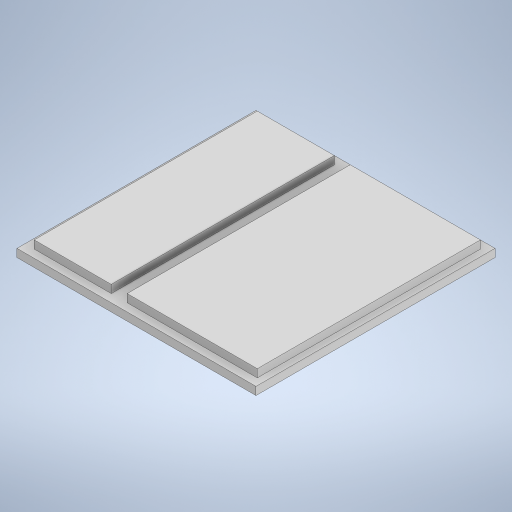
# Autodesk Inventor part: víčko
Saved by Autodesk Inventor 2024 (Build 280153000, 153)
## iProperties
Created: 2025-04-21
Part Number: víčko
Material: Všeobecné
Document SubType Name: Modeling
Designer: annav
Density: 1 g/cm^3
Appearance: Výchozí
Author: ANNA VÁVROVÁ
Autodesk Inventor part; units mm, degrees
ref_plane "YZ Plane" through (0, 0, 0) normal (1, 0, 0) x (0, 1, 0)
ref_plane "XZ Plane" through (0, 0, 0) normal (0, 1, 0) x (-1, 0, 0)
ref_plane "XY Plane" through (0, 0, 0) normal (0, 0, 1) x (1, 0, 0)
sketch "Náčrt1" plane through (0, 0, 0) normal (0, 1, 0) x (-1, 0, 0)
  line L0 (0, -63) -> (0, 63) projected
  line L1 (-63, 0) -> (63, 0) projected
  line L2 (45, 45) -> (-45, 45)
  line L3 (-45, 45) -> (-45, -45)
  line L4 (-45, -45) -> (45, -45)
  line L5 (45, -45) -> (45, 45)
  point P0 (0, 0)
  dimension "d0" = 90
  dimension "d1" = 90
  constraints: 8 end point, 2 parallel, 1 horizontal, 1 perpendicular, 2 other
  measures "d0" distance of L2.end L3.end
  measures "d1" distance between parallel lines of L3 L5
extrude "Vysunutí1" add sketch "Náčrt1" along normal blind 3
sketch "Náčrt2" plane through (0, 3, 0) normal (0, 1, 0) x (1, 0, 0)
  line L0 (0, 63) -> (0, -63) projected
  line L1 (63, 0) -> (-63, 0) projected
  line L2 (-41.5, -42) -> (-12.5, -42)
  line L3 (-12.5, -42) -> (-12.5, 42)
  line L4 (-12.5, 42) -> (-41.5, 42)
  line L5 (-41.5, 42) -> (-41.5, -42)
  line L6 (-45, 45) -> (-45, -45) projected
  point P0 (0, 0)
  dimension "d4" = 3.5
  dimension "d5" = 29
  dimension "d6" = 84
  constraints: 8 end point, 2 parallel, 1 horizontal, 1 perpendicular, 1 other
  measures "d4" distance between parallel lines of L5 L6
  measures "d5" distance between parallel lines of L3 L5
  measures "d6" distance between parallel lines of L4 L2
extrude "Vysunutí2" add sketch "Náčrt2" along normal blind 3
sketch "Náčrt3" plane through (0, 3, 0) normal (0, 1, 0) x (1, 0, 0)
  line L0 (-12.5, -42) -> (-12.5, 42) projected
  line L1 (0, 63) -> (0, -63) projected
  line L2 (63, 0) -> (-63, 0) projected
  line L3 (-6.5, -42) -> (42.5, -42)
  line L4 (42.5, -42) -> (42.5, 42)
  line L5 (42.5, 42) -> (-6.5, 42)
  line L6 (-6.5, 42) -> (-6.5, -42)
  point P0 (0, 0)
  point P1 (18, -42)
  dimension "d9" = 6
  dimension "d10" = 49
  dimension "d11" = 84
  constraints: 8 end point, 2 parallel, 1 horizontal, 1 midpoint, 1 perpendicular, 1 other
  measures "d9" distance between parallel lines of L6 L0
  measures "d10" distance of L4.end L5.end
  measures "d11" distance from line of L5 point (18, -42)
extrude "Vysunutí3" add sketch "Náčrt3" along normal blind 3
sketch "Náčrt6" plane through (0, 0, 0) normal (0, -1, 0) x (1, 0, 0)
  line L0 (0, 63) -> (0, -63) projected
  line L1 (-63, 0) -> (63, 0) projected
  line L2 (-10, 0) -> (10, 0) construction
  line L3 (-6.5, -42) -> (-6.5, 42) projected
  line L4 (-10, -2.5) -> (10, -2.5)
  line L5 (10, 2.5) -> (-10, 2.5)
  arc A0 (-10, 2.5) -> (-10, -2.5) centre (-10, 0) ccw
  arc A1 (10, -2.5) -> (10, 2.5) centre (10, 0) ccw
  point P0 (0, 0)
  point P1 (0, 0)
  dimension "d14" = 20
  dimension "d15" = 5
  constraints: 8 end point, 4 point on circle, 4 tangent, 2 centre point, 1 midpoint, 1 parallel, 1 perpendicular, 2 other
  measures "d14" distance of L2.end L2.start
  measures "d15" distance between parallel lines of L4 L5
extrude "Vysunutí4" add sketch "Náčrt6" along normal blind 5
